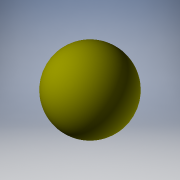
# Autodesk Inventor part: SKF_623-2RS1_ball1
Saved by Autodesk Inventor 2019 (Build 230136000, 136)
## iProperties
Created: 2023-07-31
Part Number: SKF_623-2RS1_ball1
Material: Generic
Catalog Web Link: www.cadenas.de
Description: BB1_001_101_ball1-Deep groove ball bearings
Vendor: SKF
Document SubType Name: Modeling
Designer: psAdmin
Manufacturer: SKF
Mass: 0.00209677 g
Surface Area: 0.0792229 cm^2
Volume: 0.00209677 cm^3
Density: 1 g/cm^3
Appearance: PSOLRGB-175-175-175
Category: PARTsolutions
Company: SKF
Title: SKF_623-2RS1_ball1
Author: Cadenas PARTsolutions
Comments: Deep groove ball bearings
PSOL_IDENT_0: {$CADENAS_DATA/23d-libs/skf/bearings_units_and_housings/ball_bearings/deep_groove_ball_bearings/part
PSOL_IDENT_1: s/bb1_001_101_ball1.prj},190 {VTYP=3D},{NB=SKF_623-2RS1_ball1},{LINA=SKF_623-2RS1_ball1},{NN=BB1_001
PSOL_IDENT_2: _101_ball1},{DATE=25.11.2022 05:56:16},{GEOMDATE=21.11.2022 11:35:00},{VERSION=},{LINEID=11110},{WBV
PSOL_IDENT_3: AR=},{WBNUMERIC=}  {NB=SKF_623-2RS1_ball1},{LINA=SKF_623-2RS1_ball1},{KT=DUMMY},{DESIGNATION=623-2RS
PSOL_IDENT_4: 1},{R12=0.15},{DD=3.000},{D=10.000},{B=4.000},{C=},{CX=},{CXX=},{CA=0.000},{XXVARIANT=},{XXDESIGN=Si
PSOL_IDENT_5: ngle row},{XXSEALING=Contact seal on both sides},{DESIGN=dgbbrs},{DESIGNIR=dgbbrs},{VARIANT=},{DD1=4
PSOL_IDENT_6: .80},{DD2=},{DD2X=},{DD2A=0.00},{D1=7.08},{D1X=0.00},{D2=8.2},{D2A=8.20},{D3=},{D3X=},{D3A=0.000},{D
PSOL_IDENT_7: 4=},{HH=0.000},{BB=0.000},{BBX=},{BBA=0.000},{FF=},{R0MAX=0.000},{R0=0.000},{PITCH=5.94},{DW=1.588},
PSOL_IDENT_8: {DDAMIN=4.200},{DDAMAX=5.100},{DDBMIN=0.000},{DDBMAX=0.000},{DBMIN=0.000},{DAMAX=8.800},{BBAMIN=0.00
PSOL_IDENT_9: 0},{CAMAX=0.000},{RAMAX=0.100},{LOAD1=0.540},{LOAD2=0.180},{LOAD3=0.007},{SPEED1=0},{SPEED2=40000},{
PSOL_IDENT_10: KR=0.025},{F0=7.500},{Z=7},{II=1},{MASS=0.002},{BEARING=623-2RS1},{RING=},{HELP=1.460},{HELP2=0.900}
PSOL_IDENT_11: ,{DD1ALG=2.400},{YALG=2.400},{PITCH1=5.940},{DW1=1.588},{YALG1=3.540},{HALG1=1.460},{SH=2.400},{CU=0
PSOL_IDENT_12: .482},{HALG=0.9},{B1=0},{SHIELDHELP=2},{D4A=0.000},{FFA=0.000},{RS1=X},{HELP3=0},{SUPPRESS=0}
NB: SKF_623-2RS1_ball1
NN: BB1_001_101_ball1
NT: Deep groove ball bearings
NBSYN: SKF_$DESIGNATION._ball1
LINA: SKF_623-2RS1_ball1
CATALOG: SKF
DESIGNATION: 623-2RS1
R12: 0.15
DD: 3
D: 10
B: 4
XXDESIGN: Single row
XXSEALING: Contact seal on both sides
DD1: 4.8
D1: 7.08
D1X: 0
D2: 8.2
HH: 0
BB: 0
R0MAX: 0
R0: 0
PITCH: 5.94
DW: 1.588
DDAMIN: 4.2
DDAMAX: 5.1
DDBMIN: 0
DDBMAX: 0
DBMIN: 0
DAMAX: 8.8
BBAMIN: 0
CAMAX: 0
RAMAX: 0.1
LOAD1: 0.54
LOAD2: 0.18
LOAD3: 0.007
SPEED1: 0
SPEED2: 40000
KR: 0.025
F0: 7.5
Z: 7
II: 1
MASS: 0.002
BEARING: 623-2RS1
HELP3: 0
SUPPRESS: 0
SUPPLIER: SKF
ARTICLENO: SKF_623-2RS1_ball1
BOMINFO: SKF_623-2RS1_ball1
CREATOR: CADENAS GmbH
Autodesk Inventor part; units mm, degrees
ref_plane "YZ Plane" through (0, 0, 0) normal (1, 0, 0) x (0, 1, 0)
ref_plane "XZ Plane" through (0, 0, 0) normal (0, 1, 0) x (-1, 0, 0)
ref_plane "XY Plane" through (0, 0, 0) normal (0, 0, 1) x (1, 0, 0)
sketch "Sketch_6" plane through (0, 0, 0) normal (0, 0, 1) x (1, 0, 0)
  line L0 (2.794, 2.97) -> (1.206, 2.97)
  arc A0 (2.794, 2.97) -> (1.206, 2.97) centre (2, 2.97) ccw
  line L1 (2.794, 2.97) -> (1.206, 2.97)
  constraints: 4 end point, 2 point on circle, 1 centre point
revolve "Revolution1" add sketch "Sketch_6" angle 360 about axis through (2.794, 2.97, 0) along (1, 0, 0)
ref_plane "ball1_XY" through (2, 2.97, 0) normal (1, 0, 0) x (0, 0, -1)
ref_plane "ball1_YZ" through (2, 2.97, 0) normal (0, 0, -1) x (0, 1, 0)
ref_plane "ball1_ZX" through (2, 2.97, 0) normal (0, 1, 0) x (1, 0, 0)
body "Solid1"
